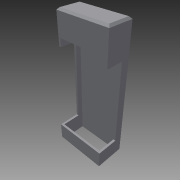
# Autodesk Inventor part: Battery Holder
Saved by Autodesk Inventor 2014 (Build 180170000, 170)
## iProperties
Created: 2014-02-28
Part Number: Battery Holder
Material: Generic
Document SubType Name: Modeling
Designer: Isaac
Density: 1 g/cm^3
Appearance: Default
Author: Isaac
Autodesk Inventor part; units mm, degrees
ref_plane "YZ Plane" through (0, 0, 0) normal (1, 0, 0) x (0, 1, 0)
ref_plane "XZ Plane" through (0, 0, 0) normal (0, 1, 0) x (-1, 0, 0)
ref_plane "XY Plane" through (0, 0, 0) normal (0, 0, 1) x (1, 0, 0)
sketch "Sketch1" plane through (0, 0, 0) normal (0, 0, 1) x (1, 0, 0)
  arc A0 (49.1564, -72.9751) -> (-49.1564, -72.9751) centre (0, -254.0664) ccw
  line L0 (49.1564, -72.9751) -> (73.0086, -49.1229)
  line L1 (86.9345, 13.6367) -> (74.7113, 47.4192)
  line L2 (74.7113, 47.4192) -> (49.163, 72.9816)
  line L3 (-49.163, 72.9816) -> (-75.1179, 47.041)
  line L4 (-75.1179, 47.041) -> (-86.9513, 13.6826)
  line L5 (-49.1564, -72.9751) -> (-73.0086, -49.1229)
  arc A1 (-49.163, 72.9816) -> (49.163, 72.9816) centre (0, 254.0664) ccw
  arc A2 (-73.0086, -49.1229) -> (-86.9513, 13.6826) centre (-146.4572, -32.478) ccw
  arc A3 (86.9345, 13.6367) -> (73.0086, -49.1229) centre (146.4645, -32.4974) ccw
  line L6 (0, 0) -> (0, -66.422)
  line L7 (0, 0) -> (0, 66.4266)
  line L8 (78.5091, -0.0284) -> (-78.4957, -0.0284)
  line L9 (-49.163, 72.9816) -> (49.163, 72.9816)
  line L10 (-49.163, 72.9816) -> (-31.7513, 72.9816)
  line L11 (-31.7513, 72.9816) -> (-31.7513, -69.1278)
  line L12 (49.163, 72.9816) -> (31.7513, 72.9816)
  line L13 (31.7513, 72.9816) -> (31.7513, -69.1278)
  line L14 (31.7513, -69.1278) -> (31.7513, 95.9722)
  line L15 (31.7513, 95.9722) -> (-31.7513, 95.9722)
  line L16 (-31.7513, 95.9722) -> (-31.7513, 72.9816)
  line L17 (31.7513, -69.1278) -> (31.7513, -81.8278)
  line L18 (31.7513, -81.8278) -> (-31.7513, -81.8278)
  line L19 (-31.7513, -81.8278) -> (-31.7513, -69.1278)
  line L20 (31.7513, 95.9722) -> (34.9263, 95.9722)
  line L21 (34.9263, 95.9722) -> (34.9263, -81.8278)
  line L22 (34.9263, -81.8278) -> (31.7513, -81.8278)
  line L23 (-31.7513, 95.9722) -> (-34.9263, 95.9722)
  line L24 (-34.9263, 95.9722) -> (-34.9263, -81.8278)
  line L25 (-34.9263, -81.8278) -> (-31.7513, -81.8278)
  line L26 (31.7513, 95.9722) -> (31.7513, 92.7972)
  line L27 (31.7513, 92.7972) -> (-31.7513, 92.7972)
  constraints: 56 end point, 14 point on circle, 10 perpendicular, 6 parallel, 5 point on line, 4 centre point, 1 collinear
extrude "Extrusion1" add sketch "Sketch1" along normal blind 3.175 contours L17 L18 L19 A0 | L13 L8 L21 A0 | A0 L6 L8 L13 | A0 L21 L22 L17 | A0 L11 L8 L6 | L13 A1 L21 L8 | L8 L6 L7 A1 L13 | L19 L25 L24 A0 | A0 L24 L8 L11 | L8 L11 A1 L7 L6 | L13 L9 L21 A1 | A1 L11 L9 L13 | L8 L24 A1 L11 | L14 L20 L21 L9 | L9 L16 L27 L14 | A1 L24 L9 L11 | L9 L24 L23 L16 | L27 L16 L15 L14
sketch "Sketch2" plane through (0, 0, 3.175) normal (0, 0, 1) x (1, 0, 0)
  line L0 (34.9263, 95.9722) -> (-34.9263, 95.9722) projected
  line L1 (-34.9263, 95.9722) -> (-34.9263, -81.8278) projected
  line L2 (-34.9263, -81.8278) -> (34.9263, -81.8278) projected
  line L3 (34.9263, -81.8278) -> (34.9263, 95.9722) projected
  line L4 (-34.9263, 95.9722) -> (-34.9263, 92.7972)
  line L5 (-34.9263, 92.7972) -> (34.9263, 92.7972)
  line L6 (34.9263, -81.8278) -> (31.7513, -81.8278)
  line L7 (31.7513, -81.8278) -> (31.7513, 92.7972)
  line L8 (-34.9263, -81.8278) -> (-31.7513, -81.8278)
  line L9 (-31.7513, -81.8278) -> (-31.7513, 92.7972)
  point P0 (0, 0)
  dimension "d9" = 3.175
  dimension "d10" = 3.175
  dimension "d11" = 3.175
  constraints: 12 end point, 6 point on line, 3 perpendicular
  measures "d9" distance of L0.end L4.end
  measures "d10" distance of L2.end L6.end
  measures "d11" distance of L1.end L8.end
extrude "Extrusion2" add sketch "Sketch2" along normal blind 28.575 contours L3 L5 L1 L0 | L3 L2 L7 L5 | L5 L9 L2 L1
sketch "Sketch3" plane through (-31.7513, 92.7972, 3.175) normal (0, -1, 0) x (1, 0, 0)
  line L0 (63.5025, 0) -> (63.5025, 28.575) projected
  line L1 (0, 28.575) -> (63.5025, 28.575) projected
  line L2 (0, 28.575) -> (0, 0) projected
  line L3 (63.5025, 28.575) -> (63.5025, 25.4)
  line L4 (63.5025, 25.4) -> (0, 25.4)
  point P0 (31.7513, -3.175)
  dimension "d14" = 3.175
  constraints: 4 end point, 2 point on line, 1 perpendicular
  measures "d14" distance of L0.end L3.end
extrude "Extrusion3" add sketch "Sketch3" along normal blind 28.575
sketch "Sketch4" plane through (34.9263, -81.8278, 0) normal (1, 0, 0) x (0, 0, -1)
  line L0 (-31.75, 0) -> (-31.75, 177.8) projected
  line L1 (0, 0) -> (-31.75, 0) projected
  line L2 (-31.75, 0) -> (-31.75, 135.5494)
  line L3 (-31.75, 135.5494) -> (-10.3194, 135.5494)
  line L4 (-10.3194, 135.5494) -> (-10.3194, 0)
  point P0 (0, 81.8278)
  constraints: 6 end point, 2 perpendicular, 2 point on line
extrude "Extrusion4" cut sketch "Sketch4" against normal blind 127
sketch "Sketch5" plane through (34.9263, -81.8278, 10.3194) normal (0, 0, 1) x (1, 0, 0)
  line L0 (-3.175, 0) -> (-3.175, 135.5494) projected
  line L1 (0, 0) -> (-3.175, 0) projected
  line L2 (0, 135.5494) -> (0, 0) projected
  line L3 (0, 0) -> (0, 25.4)
  line L4 (0, 25.4) -> (-3.175, 25.4)
  point P0 (-34.9263, 81.8278)
  dimension "d19" = 25.4
  constraints: 4 end point, 2 point on line, 1 perpendicular
  measures "d19" distance of L1.start L3.end
sketch "Sketch6" plane through (-34.9263, 53.7216, 10.3194) normal (0, 0, 1) x (1, 0, 0)
  line L0 (3.175, 0) -> (3.175, -135.5494) projected
  line L1 (0, -135.5494) -> (0, 0) projected
  line L2 (3.175, -135.5494) -> (0, -135.5494) projected
  line L3 (3.175, -135.5494) -> (3.175, -110.1494)
  line L4 (3.175, -110.1494) -> (0, -110.1494)
  point P0 (34.9263, -53.7216)
  dimension "d20" = 25.4
  constraints: 4 end point, 2 point on line, 1 perpendicular
  measures "d20" distance of L0.end L3.end
extrude "Extrusion5" add sketch "Sketch6" along normal blind 28.575
extrude "Extrusion6" add sketch "Sketch5" along normal blind 28.575
sketch "Sketch7" plane through (31.7513, -81.8278, 3.175) normal (-1, 0, 0) x (0, 0, 1)
  line L0 (0, 0) -> (35.7194, 0) projected
  line L1 (35.7194, 25.4) -> (35.7194, 0) projected
  line L2 (7.1444, 25.4) -> (35.7194, 25.4) projected
  line L3 (35.7194, 25.4) -> (32.5444, 25.4)
  line L4 (32.5444, 25.4) -> (32.5444, 0)
  point P0 (-3.175, 81.8278)
  dimension "d25" = 3.175
  constraints: 4 end point, 2 point on line, 1 perpendicular
  measures "d25" distance of L1.start L3.end
extrude "Extrusion7" add sketch "Sketch7" along normal blind 66.04
chamfer "Chamfer1" distance 2.54 angle 45 5 edges at (0, 95.9722, 31.75) (-34.9263, 95.9722, 15.875) (0, 92.7972, 3.175) (34.9263, 95.9722, 15.875) (0, 95.9722, 0)
chamfer "Chamfer2" distance 2.54 angle 45 4 edges at (0, -81.8278, 38.8944) (0, -81.8278, 0) (-34.9263, -81.8278, 19.4472) (34.9263, -81.8278, 19.4472)
body "Solid1"
